Autodesk Fusion 360 part; units mm, degrees
(part 2 of 8)
  line L971 (783.8506, -24.35) -> (783.8506, -21.35)
  line L972 (783.8506, -21.35) -> (780.8506, -21.35)
  line L973 (780.8506, -21.35) -> (780.8506, -24.35)
  line L974 (780.8506, -24.35) -> (777.8506, -24.35)
  line L975 (777.8506, -24.35) -> (777.8506, -21.35)
  line L976 (777.8506, -21.35) -> (774.8506, -21.35)
  line L977 (774.8506, -21.35) -> (774.8506, -24.35)
  line L978 (774.8506, -24.35) -> (771.8506, -24.35)
  line L979 (771.8506, -24.35) -> (771.8506, -21.35)
  line L980 (771.8506, -21.35) -> (768.8506, -21.35)
  line L981 (768.8506, -21.35) -> (768.8506, -24.35)
  line L982 (768.8506, -24.35) -> (765.8506, -24.35)
  line L983 (765.8506, -24.35) -> (765.8506, -21.35)
  line L984 (765.8506, -21.35) -> (762.8506, -21.35)
  line L985 (762.8506, -21.35) -> (762.8506, -24.35)
  line L986 (762.8506, -24.35) -> (759.8506, -24.35)
  line L987 (759.8506, -24.35) -> (759.8506, -21.35)
  line L988 (759.8506, -21.35) -> (756.8506, -21.35)
  line L989 (756.8506, -21.35) -> (756.8506, -24.35)
  line L990 (756.8506, -24.35) -> (753.8506, -24.35)
  line L991 (753.8506, -24.35) -> (753.8506, -21.35)
  line L992 (753.8506, -21.35) -> (750.8506, -21.35)
  line L993 (750.8506, -21.35) -> (750.8506, -24.35)
  line L994 (750.8506, -24.35) -> (747.8506, -24.35)
  line L995 (747.8506, -24.35) -> (747.8506, -21.35)
  line L996 (747.8506, -21.35) -> (744.8506, -21.35)
  line L997 (744.8506, -21.35) -> (744.8506, -24.35)
  line L998 (744.8506, -24.35) -> (741.8506, -24.35)
  line L999 (741.8506, -24.35) -> (741.8506, -21.35)
  line L1000 (741.8506, -21.35) -> (738.8506, -21.35)
  line L1001 (738.8506, -21.35) -> (738.8506, -24.35)
  line L1002 (738.8506, -24.35) -> (735.8506, -24.35)
  line L1003 (735.8506, -24.35) -> (735.8506, -21.35)
  line L1004 (735.8506, -21.35) -> (732.8506, -21.35)
  line L1005 (732.8506, -21.35) -> (732.8506, -24.35)
  line L1006 (732.8506, -24.35) -> (729.8506, -24.35)
  line L1007 (729.8506, -24.35) -> (729.8506, -21.35)
  line L1008 (729.8506, -21.35) -> (726.8506, -21.35)
  line L1009 (726.8506, -21.35) -> (726.8506, -24.35)
  line L1010 (726.8506, -24.35) -> (723.8506, -24.35)
  line L1011 (723.8506, -24.35) -> (723.8506, -21.35)
  line L1012 (723.8506, -21.35) -> (720.8506, -21.35)
  line L1013 (720.8506, -21.35) -> (720.8506, -24.35)
  line L1014 (720.8506, -24.35) -> (717.8506, -24.35)
  line L1015 (717.8506, -24.35) -> (717.8506, -21.35)
  line L1016 (717.8506, -21.35) -> (714.8506, -21.35)
  line L1017 (714.8506, -21.35) -> (714.8506, -24.35)
  line L1018 (714.8506, -24.35) -> (711.8506, -24.35)
  line L1019 (711.8506, -24.35) -> (711.8506, -21.35)
  line L1020 (711.8506, -21.35) -> (708.8506, -21.35)
  line L1021 (708.8506, -21.35) -> (708.8506, -24.35)
  line L1022 (708.8506, -24.35) -> (705.8506, -24.35)
  line L1023 (705.8506, -24.35) -> (705.8506, -21.35)
  line L1024 (705.8506, -21.35) -> (702.8506, -21.35)
  line L1025 (702.8506, -21.35) -> (702.8506, -24.35)
  line L1026 (702.8506, -24.35) -> (699.8506, -24.35)
  line L1027 (699.8506, -24.35) -> (699.8506, -21.35)
  line L1028 (699.8506, -21.35) -> (696.8506, -21.35)
  line L1029 (696.8506, -21.35) -> (696.8506, -24.35)
  line L1030 (696.8506, -24.35) -> (693.8506, -24.35)
  line L1031 (693.8506, -24.35) -> (693.8506, -21.35)
  line L1032 (693.8506, -21.35) -> (690.8506, -21.35)
  line L1033 (690.8506, -21.35) -> (690.8506, -24.35)
  line L1034 (690.8506, -24.35) -> (687.8506, -24.35)
  line L1035 (687.8506, -24.35) -> (687.8506, -21.35)
  line L1036 (687.8506, -21.35) -> (684.8506, -21.35)
  line L1037 (684.8506, -21.35) -> (684.8506, -24.35)
  line L1038 (684.8506, -24.35) -> (681.8506, -24.35)
  line L1039 (681.8506, -24.35) -> (681.8506, -21.35)
  line L1040 (681.8506, -21.35) -> (678.8506, -21.35)
  line L1041 (678.8506, -21.35) -> (678.8506, -24.35)
  line L1042 (678.8506, -24.35) -> (675.8506, -24.35)
  line L1043 (675.8506, -24.35) -> (675.8506, -21.35)
  line L1044 (675.8506, -21.35) -> (672.8506, -21.35)
  line L1045 (672.8506, -21.35) -> (672.8506, -24.35)
  line L1046 (672.8506, -24.35) -> (669.8506, -24.35)
  line L1047 (669.8506, -24.35) -> (669.8506, -21.35)
  line L1048 (669.8506, -21.35) -> (666.8505, -21.35)
  line L1049 (666.8505, -21.35) -> (666.8505, -24.35)
  line L1050 (666.8505, -24.35) -> (663.8505, -24.35)
  line L1051 (663.8505, -24.35) -> (663.8505, -21.35)
  line L1052 (663.8505, -21.35) -> (660.8505, -21.35)
  line L1053 (660.8505, -21.35) -> (660.8505, -24.35)
  line L1054 (660.8505, -24.35) -> (657.8505, -24.35)
  line L1055 (657.8505, -24.35) -> (657.8505, -21.35)
  line L1056 (657.8505, -21.35) -> (654.8505, -21.35)
  line L1057 (654.8505, -21.35) -> (654.8505, -24.35)
  line L1058 (654.8505, -24.35) -> (651.8505, -24.35)
  line L1059 (651.8505, -24.35) -> (651.8505, -21.35)
  line L1060 (651.8505, -21.35) -> (648.8505, -21.35)
  line L1061 (648.8505, -21.35) -> (648.8505, -24.35)
  line L1062 (648.8505, -24.35) -> (645.8505, -24.35)
  line L1063 (645.8505, -24.35) -> (645.8505, -21.35)
  line L1064 (645.8505, -21.35) -> (642.1005, -21.35)
  line L1065 (642.1005, -21.35) -> (642.1005, -24.35)
  line L1066 (642.1005, -24.35) -> (641.3505, -24.35)
  line L1067 (641.3505, -24.35) -> (641.3505, -20.6)
  line L1068 (641.3505, -20.6) -> (638.3505, -20.6)
  line L1069 (638.3505, -20.6) -> (638.3505, -16.85)
  line L1070 (638.3505, -16.85) -> (641.3505, -16.85)
  line L1071 (641.3505, -16.85) -> (641.3505, -13.85)
  line L1072 (641.3505, -13.85) -> (638.3505, -13.85)
  line L1073 (638.3505, -13.85) -> (638.3505, -10.1)
  line L1074 (638.3505, -10.1) -> (641.3505, -10.1)
  line L1075 (641.3505, -10.1) -> (641.3505, -6.35)
  line L1076 (641.3505, -24.35) -> (642.1005, -24.35)
  line L1077 (642.1005, -24.35) -> (642.1005, -27.35)
  line L1078 (642.1005, -27.35) -> (645.8505, -27.35)
  line L1079 (645.8505, -27.35) -> (645.8505, -24.35)
  line L1080 (645.8505, -24.35) -> (648.8505, -24.35)
  line L1081 (648.8505, -24.35) -> (648.8505, -27.35)
  line L1082 (648.8505, -27.35) -> (651.8505, -27.35)
  line L1083 (651.8505, -27.35) -> (651.8505, -24.35)
  line L1084 (651.8505, -24.35) -> (654.8505, -24.35)
  line L1085 (654.8505, -24.35) -> (654.8505, -27.35)
  line L1086 (654.8505, -27.35) -> (657.8505, -27.35)
  line L1087 (657.8505, -27.35) -> (657.8505, -24.35)
  line L1088 (657.8505, -24.35) -> (660.8505, -24.35)
  line L1089 (660.8505, -24.35) -> (660.8505, -27.35)
  line L1090 (660.8505, -27.35) -> (663.8505, -27.35)
  line L1091 (663.8505, -27.35) -> (663.8505, -24.35)
  line L1092 (663.8505, -24.35) -> (666.8505, -24.35)
  line L1093 (666.8505, -24.35) -> (666.8505, -27.35)
  line L1094 (666.8505, -27.35) -> (669.8506, -27.35)
  line L1095 (669.8506, -27.35) -> (669.8506, -24.35)
  line L1096 (669.8506, -24.35) -> (672.8506, -24.35)
  line L1097 (672.8506, -24.35) -> (672.8506, -27.35)
  line L1098 (672.8506, -27.35) -> (675.8506, -27.35)
  line L1099 (675.8506, -27.35) -> (675.8506, -24.35)
  line L1100 (675.8506, -24.35) -> (678.8506, -24.35)
  line L1101 (678.8506, -24.35) -> (678.8506, -27.35)
  line L1102 (678.8506, -27.35) -> (681.8506, -27.35)
  line L1103 (681.8506, -27.35) -> (681.8506, -24.35)
  line L1104 (681.8506, -24.35) -> (684.8506, -24.35)
  line L1105 (684.8506, -24.35) -> (684.8506, -27.35)
  line L1106 (684.8506, -27.35) -> (687.8506, -27.35)
  line L1107 (687.8506, -27.35) -> (687.8506, -24.35)
  line L1108 (687.8506, -24.35) -> (690.8506, -24.35)
  line L1109 (690.8506, -24.35) -> (690.8506, -27.35)
  line L1110 (690.8506, -27.35) -> (693.8506, -27.35)
  line L1111 (693.8506, -27.35) -> (693.8506, -24.35)
  line L1112 (693.8506, -24.35) -> (696.8506, -24.35)
  line L1113 (696.8506, -24.35) -> (696.8506, -27.35)
  line L1114 (696.8506, -27.35) -> (699.8506, -27.35)
  line L1115 (699.8506, -27.35) -> (699.8506, -24.35)
  line L1116 (699.8506, -24.35) -> (702.8506, -24.35)
  line L1117 (702.8506, -24.35) -> (702.8506, -27.35)
  line L1118 (702.8506, -27.35) -> (705.8506, -27.35)
  line L1119 (705.8506, -27.35) -> (705.8506, -24.35)
  line L1120 (705.8506, -24.35) -> (708.8506, -24.35)
  line L1121 (708.8506, -24.35) -> (708.8506, -27.35)
  line L1122 (708.8506, -27.35) -> (711.8506, -27.35)
  line L1123 (711.8506, -27.35) -> (711.8506, -24.35)
  line L1124 (711.8506, -24.35) -> (714.8506, -24.35)
  line L1125 (714.8506, -24.35) -> (714.8506, -27.35)
  line L1126 (714.8506, -27.35) -> (717.8506, -27.35)
  line L1127 (717.8506, -27.35) -> (717.8506, -24.35)
  line L1128 (717.8506, -24.35) -> (720.8506, -24.35)
  line L1129 (720.8506, -24.35) -> (720.8506, -27.35)
  line L1130 (720.8506, -27.35) -> (723.8506, -27.35)
  line L1131 (723.8506, -27.35) -> (723.8506, -24.35)
  line L1132 (723.8506, -24.35) -> (726.8506, -24.35)
  line L1133 (726.8506, -24.35) -> (726.8506, -27.35)
  line L1134 (726.8506, -27.35) -> (729.8506, -27.35)
  line L1135 (729.8506, -27.35) -> (729.8506, -24.35)
  line L1136 (729.8506, -24.35) -> (732.8506, -24.35)
  line L1137 (732.8506, -24.35) -> (732.8506, -27.35)
  line L1138 (732.8506, -27.35) -> (735.8506, -27.35)
  line L1139 (735.8506, -27.35) -> (735.8506, -24.35)
  line L1140 (735.8506, -24.35) -> (738.8506, -24.35)
  line L1141 (738.8506, -24.35) -> (738.8506, -27.35)
  line L1142 (738.8506, -27.35) -> (741.8506, -27.35)
  line L1143 (741.8506, -27.35) -> (741.8506, -24.35)
  line L1144 (741.8506, -24.35) -> (744.8506, -24.35)
  line L1145 (744.8506, -24.35) -> (744.8506, -27.35)
  line L1146 (744.8506, -27.35) -> (747.8506, -27.35)
  line L1147 (747.8506, -27.35) -> (747.8506, -24.35)
  line L1148 (747.8506, -24.35) -> (750.8506, -24.35)
  line L1149 (750.8506, -24.35) -> (750.8506, -27.35)
  line L1150 (750.8506, -27.35) -> (753.8506, -27.35)
  line L1151 (753.8506, -27.35) -> (753.8506, -24.35)
  line L1152 (753.8506, -24.35) -> (756.8506, -24.35)
  line L1153 (756.8506, -24.35) -> (756.8506, -27.35)
  line L1154 (756.8506, -27.35) -> (759.8506, -27.35)
  line L1155 (759.8506, -27.35) -> (759.8506, -24.35)
  line L1156 (759.8506, -24.35) -> (762.8506, -24.35)
  line L1157 (762.8506, -24.35) -> (762.8506, -27.35)
  line L1158 (762.8506, -27.35) -> (765.8506, -27.35)
  line L1159 (765.8506, -27.35) -> (765.8506, -24.35)
  line L1160 (765.8506, -24.35) -> (768.8506, -24.35)
  line L1161 (768.8506, -24.35) -> (768.8506, -27.35)
  line L1162 (768.8506, -27.35) -> (771.8506, -27.35)
  line L1163 (771.8506, -27.35) -> (771.8506, -24.35)
  line L1164 (771.8506, -24.35) -> (774.8506, -24.35)
  line L1165 (774.8506, -24.35) -> (774.8506, -27.35)
  line L1166 (774.8506, -27.35) -> (777.8506, -27.35)
  line L1167 (777.8506, -27.35) -> (777.8506, -24.35)
  line L1168 (777.8506, -24.35) -> (780.8506, -24.35)
  line L1169 (780.8506, -24.35) -> (780.8506, -27.35)
  line L1170 (780.8506, -27.35) -> (783.8506, -27.35)
  line L1171 (783.8506, -27.35) -> (783.8506, -24.35)
  line L1172 (783.8506, -24.35) -> (786.8506, -24.35)
  line L1173 (786.8506, -24.35) -> (786.8506, -27.35)
  line L1174 (786.8506, -27.35) -> (790.6007, -27.35)
  line L1175 (790.6007, -27.35) -> (790.6007, -24.35)
  line L1176 (790.6007, -24.35) -> (791.3507, -24.35)
  line L1177 (791.3507, -24.35) -> (791.3507, -28.1)
  line L1178 (791.3507, -28.1) -> (794.3507, -28.1)
  line L1179 (794.3507, -28.1) -> (794.3507, -31.85)
  line L1180 (794.3507, -31.85) -> (791.3507, -31.85)
  line L1181 (791.3507, -31.85) -> (791.3507, -34.85)
  line L1182 (791.3507, -34.85) -> (794.3507, -34.85)
  line L1183 (794.3507, -34.85) -> (794.3507, -38.6)
  line L1184 (794.3507, -38.6) -> (791.3507, -38.6)
  line L1185 (791.3507, -38.6) -> (791.3507, -42.35)
  line L1186 (791.3507, -42.35) -> (790.6007, -42.35)
  line L1187 (790.6007, -42.35) -> (790.6007, -39.35)
  line L1188 (790.6007, -39.35) -> (786.8506, -39.35)
  line L1189 (786.8506, -39.35) -> (786.8506, -42.35)
  line L1190 (786.8506, -42.35) -> (783.8506, -42.35)
  line L1191 (783.8506, -42.35) -> (783.8506, -39.35)
  line L1192 (783.8506, -39.35) -> (780.8506, -39.35)
  line L1193 (780.8506, -39.35) -> (780.8506, -42.35)
  line L1194 (780.8506, -42.35) -> (777.8506, -42.35)
  line L1195 (777.8506, -42.35) -> (777.8506, -39.35)
  line L1196 (777.8506, -39.35) -> (774.8506, -39.35)
  line L1197 (774.8506, -39.35) -> (774.8506, -42.35)
  line L1198 (774.8506, -42.35) -> (771.8506, -42.35)
  line L1199 (771.8506, -42.35) -> (771.8506, -39.35)
  line L1200 (771.8506, -39.35) -> (768.8506, -39.35)
  line L1201 (768.8506, -39.35) -> (768.8506, -42.35)
  line L1202 (768.8506, -42.35) -> (765.8506, -42.35)
  line L1203 (765.8506, -42.35) -> (765.8506, -39.35)
  line L1204 (765.8506, -39.35) -> (762.8506, -39.35)
  line L1205 (762.8506, -39.35) -> (762.8506, -42.35)
  line L1206 (762.8506, -42.35) -> (759.8506, -42.35)
  line L1207 (759.8506, -42.35) -> (759.8506, -39.35)
  line L1208 (759.8506, -39.35) -> (756.8506, -39.35)
  line L1209 (756.8506, -39.35) -> (756.8506, -42.35)
  line L1210 (756.8506, -42.35) -> (753.8506, -42.35)
  line L1211 (753.8506, -42.35) -> (753.8506, -39.35)
  line L1212 (753.8506, -39.35) -> (750.8506, -39.35)
  line L1213 (750.8506, -39.35) -> (750.8506, -42.35)
  line L1214 (750.8506, -42.35) -> (747.8506, -42.35)
  line L1215 (747.8506, -42.35) -> (747.8506, -39.35)
  line L1216 (747.8506, -39.35) -> (744.8506, -39.35)
  line L1217 (744.8506, -39.35) -> (744.8506, -42.35)
  line L1218 (744.8506, -42.35) -> (741.8506, -42.35)
  line L1219 (741.8506, -42.35) -> (741.8506, -39.35)
  line L1220 (741.8506, -39.35) -> (738.8506, -39.35)
  line L1221 (738.8506, -39.35) -> (738.8506, -42.35)
  line L1222 (738.8506, -42.35) -> (735.8506, -42.35)
  line L1223 (735.8506, -42.35) -> (735.8506, -39.35)
  line L1224 (735.8506, -39.35) -> (732.8506, -39.35)
  line L1225 (732.8506, -39.35) -> (732.8506, -42.35)
  line L1226 (732.8506, -42.35) -> (729.8506, -42.35)
  line L1227 (729.8506, -42.35) -> (729.8506, -39.35)
  line L1228 (729.8506, -39.35) -> (726.8506, -39.35)
  line L1229 (726.8506, -39.35) -> (726.8506, -42.35)
  line L1230 (726.8506, -42.35) -> (723.8506, -42.35)
  line L1231 (723.8506, -42.35) -> (723.8506, -39.35)
  line L1232 (723.8506, -39.35) -> (720.8506, -39.35)
  line L1233 (720.8506, -39.35) -> (720.8506, -42.35)
  line L1234 (720.8506, -42.35) -> (717.8506, -42.35)
  line L1235 (717.8506, -42.35) -> (717.8506, -39.35)
  line L1236 (717.8506, -39.35) -> (714.8506, -39.35)
  line L1237 (714.8506, -39.35) -> (714.8506, -42.35)
  line L1238 (714.8506, -42.35) -> (711.8506, -42.35)
  line L1239 (711.8506, -42.35) -> (711.8506, -39.35)
  line L1240 (711.8506, -39.35) -> (708.8506, -39.35)
  line L1241 (708.8506, -39.35) -> (708.8506, -42.35)
  line L1242 (708.8506, -42.35) -> (705.8506, -42.35)
  line L1243 (705.8506, -42.35) -> (705.8506, -39.35)
  line L1244 (705.8506, -39.35) -> (702.8506, -39.35)
  line L1245 (702.8506, -39.35) -> (702.8506, -42.35)
  line L1246 (702.8506, -42.35) -> (699.8506, -42.35)
  line L1247 (699.8506, -42.35) -> (699.8506, -39.35)
  line L1248 (699.8506, -39.35) -> (696.8506, -39.35)
  line L1249 (696.8506, -39.35) -> (696.8506, -42.35)
  line L1250 (696.8506, -42.35) -> (693.8506, -42.35)
  line L1251 (693.8506, -42.35) -> (693.8506, -39.35)
  line L1252 (693.8506, -39.35) -> (690.8506, -39.35)
  line L1253 (690.8506, -39.35) -> (690.8506, -42.35)
  line L1254 (690.8506, -42.35) -> (687.8506, -42.35)
  line L1255 (687.8506, -42.35) -> (687.8506, -39.35)
  line L1256 (687.8506, -39.35) -> (684.8506, -39.35)
  line L1257 (684.8506, -39.35) -> (684.8506, -42.35)
  line L1258 (684.8506, -42.35) -> (681.8506, -42.35)
  line L1259 (681.8506, -42.35) -> (681.8506, -39.35)
  line L1260 (681.8506, -39.35) -> (678.8506, -39.35)
  line L1261 (678.8506, -39.35) -> (678.8506, -42.35)
  line L1262 (678.8506, -42.35) -> (675.8506, -42.35)
  line L1263 (675.8506, -42.35) -> (675.8506, -39.35)
  line L1264 (675.8506, -39.35) -> (672.8506, -39.35)
  line L1265 (672.8506, -39.35) -> (672.8506, -42.35)
  line L1266 (672.8506, -42.35) -> (669.8506, -42.35)
  line L1267 (669.8506, -42.35) -> (669.8506, -39.35)
  line L1268 (669.8506, -39.35) -> (666.8505, -39.35)
  line L1269 (666.8505, -39.35) -> (666.8505, -42.35)
  line L1270 (666.8505, -42.35) -> (663.8505, -42.35)
  line L1271 (663.8505, -42.35) -> (663.8505, -39.35)
  line L1272 (663.8505, -39.35) -> (660.8505, -39.35)
  line L1273 (660.8505, -39.35) -> (660.8505, -42.35)
  line L1274 (660.8505, -42.35) -> (657.8505, -42.35)
  line L1275 (657.8505, -42.35) -> (657.8505, -39.35)
  line L1276 (657.8505, -39.35) -> (654.8505, -39.35)
  line L1277 (654.8505, -39.35) -> (654.8505, -42.35)
  line L1278 (654.8505, -42.35) -> (651.8505, -42.35)
  line L1279 (651.8505, -42.35) -> (651.8505, -39.35)
  line L1280 (651.8505, -39.35) -> (648.8505, -39.35)
  line L1281 (648.8505, -39.35) -> (648.8505, -42.35)
  line L1282 (648.8505, -42.35) -> (645.8505, -42.35)
  line L1283 (645.8505, -42.35) -> (645.8505, -39.35)
  line L1284 (645.8505, -39.35) -> (642.1005, -39.35)
  line L1285 (642.1005, -39.35) -> (642.1005, -42.35)
  line L1286 (642.1005, -42.35) -> (641.3505, -42.35)
  line L1287 (641.3505, -42.35) -> (641.3505, -38.6)
  line L1288 (641.3505, -38.6) -> (638.3505, -38.6)
  line L1289 (638.3505, -38.6) -> (638.3505, -34.85)
  line L1290 (638.3505, -34.85) -> (641.3505, -34.85)
  line L1291 (641.3505, -34.85) -> (641.3505, -31.85)
  line L1292 (641.3505, -31.85) -> (638.3505, -31.85)
  line L1293 (638.3505, -31.85) -> (638.3505, -28.1)
  line L1294 (638.3505, -28.1) -> (641.3505, -28.1)
  line L1295 (641.3505, -28.1) -> (641.3505, -24.35)
  line L1296 (9.35, -27.35) -> (11.1, -27.35)
  line L1297 (11.1, -27.35) -> (11.1, -24.35)
  line L1298 (11.1, -24.35) -> (15.85, -24.35)
  line L1299 (15.85, -24.35) -> (15.85, -27.35)
  line L1300 (15.85, -27.35) -> (18.85, -27.35)
  line L1301 (18.85, -27.35) -> (18.85, -24.35)
  line L1302 (18.85, -24.35) -> (21.85, -24.35)
  line L1303 (21.85, -24.35) -> (21.85, -27.35)
  line L1304 (21.85, -27.35) -> (24.85, -27.35)
  line L1305 (24.85, -27.35) -> (24.85, -24.35)
  line L1306 (24.85, -24.35) -> (27.85, -24.35)
  line L1307 (27.85, -24.35) -> (27.85, -27.35)
  line L1308 (27.85, -27.35) -> (30.85, -27.35)
  line L1309 (30.85, -27.35) -> (30.85, -24.35)
  line L1310 (30.85, -24.35) -> (33.85, -24.35)
  line L1311 (33.85, -24.35) -> (33.85, -27.35)
  line L1312 (33.85, -27.35) -> (36.85, -27.35)
  line L1313 (36.85, -27.35) -> (36.85, -24.35)
  line L1314 (36.85, -24.35) -> (39.85, -24.35)
  line L1315 (39.85, -24.35) -> (39.85, -27.35)
  line L1316 (39.85, -27.35) -> (42.85, -27.35)
  line L1317 (42.85, -27.35) -> (42.85, -24.35)
  line L1318 (42.85, -24.35) -> (45.85, -24.35)
  line L1319 (45.85, -24.35) -> (45.85, -27.35)
  line L1320 (45.85, -27.35) -> (48.85, -27.35)
  line L1321 (48.85, -27.35) -> (48.85, -24.35)
  line L1322 (48.85, -24.35) -> (51.85, -24.35)
  line L1323 (51.85, -24.35) -> (51.85, -27.35)
  line L1324 (51.85, -27.35) -> (54.85, -27.35)
  line L1325 (54.85, -27.35) -> (54.85, -24.35)
  line L1326 (54.85, -24.35) -> (57.85, -24.35)
  line L1327 (57.85, -24.35) -> (57.85, -27.35)
  line L1328 (57.85, -27.35) -> (60.8501, -27.35)
  line L1329 (60.8501, -27.35) -> (60.8501, -24.35)
  line L1330 (60.8501, -24.35) -> (63.8501, -24.35)
  line L1331 (63.8501, -24.35) -> (63.8501, -27.35)
  line L1332 (63.8501, -27.35) -> (66.8501, -27.35)
  line L1333 (66.8501, -27.35) -> (66.8501, -24.35)
  line L1334 (66.8501, -24.35) -> (69.8501, -24.35)
  line L1335 (69.8501, -24.35) -> (69.8501, -27.35)
  line L1336 (69.8501, -27.35) -> (72.8501, -27.35)
  line L1337 (72.8501, -27.35) -> (72.8501, -24.35)
  line L1338 (72.8501, -24.35) -> (75.8501, -24.35)
  line L1339 (75.8501, -24.35) -> (75.8501, -27.35)
  line L1340 (75.8501, -27.35) -> (78.8501, -27.35)
  line L1341 (78.8501, -27.35) -> (78.8501, -24.35)
  line L1342 (78.8501, -24.35) -> (81.8501, -24.35)
  line L1343 (81.8501, -24.35) -> (81.8501, -27.35)
  line L1344 (81.8501, -27.35) -> (84.8501, -27.35)
  line L1345 (84.8501, -27.35) -> (84.8501, -24.35)
  line L1346 (84.8501, -24.35) -> (87.8501, -24.35)
  line L1347 (87.8501, -24.35) -> (87.8501, -27.35)
  line L1348 (87.8501, -27.35) -> (90.8501, -27.35)
  line L1349 (90.8501, -27.35) -> (90.8501, -24.35)
  line L1350 (90.8501, -24.35) -> (93.8501, -24.35)
  line L1351 (93.8501, -24.35) -> (93.8501, -27.35)
  line L1352 (93.8501, -27.35) -> (96.8501, -27.35)
  line L1353 (96.8501, -27.35) -> (96.8501, -24.35)
  line L1354 (96.8501, -24.35) -> (99.8501, -24.35)
  line L1355 (99.8501, -24.35) -> (99.8501, -27.35)
  line L1356 (99.8501, -27.35) -> (102.8501, -27.35)
  line L1357 (102.8501, -27.35) -> (102.8501, -24.35)
  line L1358 (102.8501, -24.35) -> (105.8501, -24.35)
  line L1359 (105.8501, -24.35) -> (105.8501, -27.35)
  line L1360 (105.8501, -27.35) -> (108.8501, -27.35)
  line L1361 (108.8501, -27.35) -> (108.8501, -24.35)
  line L1362 (108.8501, -24.35) -> (111.8501, -24.35)
  line L1363 (111.8501, -24.35) -> (111.8501, -27.35)
  line L1364 (111.8501, -27.35) -> (114.8501, -27.35)
  line L1365 (114.8501, -27.35) -> (114.8501, -24.35)
  line L1366 (114.8501, -24.35) -> (117.8501, -24.35)
  line L1367 (117.8501, -24.35) -> (117.8501, -27.35)
  line L1368 (117.8501, -27.35) -> (120.8501, -27.35)
  line L1369 (120.8501, -27.35) -> (120.8501, -24.35)
  line L1370 (120.8501, -24.35) -> (123.8501, -24.35)
  line L1371 (123.8501, -24.35) -> (123.8501, -27.35)
  line L1372 (123.8501, -27.35) -> (126.8501, -27.35)
  line L1373 (126.8501, -27.35) -> (126.8501, -24.35)
  line L1374 (126.8501, -24.35) -> (129.8501, -24.35)
  line L1375 (129.8501, -24.35) -> (129.8501, -27.35)
  line L1376 (129.8501, -27.35) -> (132.8501, -27.35)
  line L1377 (132.8501, -27.35) -> (132.8501, -24.35)
  line L1378 (132.8501, -24.35) -> (135.8501, -24.35)
  line L1379 (135.8501, -24.35) -> (135.8501, -27.35)
  line L1380 (135.8501, -27.35) -> (138.8501, -27.35)
  line L1381 (138.8501, -27.35) -> (138.8501, -24.35)
  line L1382 (138.8501, -24.35) -> (141.8501, -24.35)
  line L1383 (141.8501, -24.35) -> (141.8501, -27.35)
  line L1384 (141.8501, -27.35) -> (144.8501, -27.35)
  line L1385 (144.8501, -27.35) -> (144.8501, -24.35)
  line L1386 (144.8501, -24.35) -> (147.8501, -24.35)
  line L1387 (147.8501, -24.35) -> (147.8501, -27.35)
  line L1388 (147.8501, -27.35) -> (150.8501, -27.35)
  line L1389 (150.8501, -27.35) -> (150.8501, -24.35)
  line L1390 (150.8501, -24.35) -> (153.8501, -24.35)
  line L1391 (153.8501, -24.35) -> (153.8501, -27.35)
  line L1392 (153.8501, -27.35) -> (156.8501, -27.35)
  line L1393 (156.8501, -27.35) -> (156.8501, -24.35)
  line L1394 (156.8501, -24.35) -> (159.8501, -24.35)
  line L1395 (159.8501, -24.35) -> (159.8501, -27.35)
  line L1396 (159.8501, -27.35) -> (162.8501, -27.35)
  line L1397 (162.8501, -27.35) -> (162.8501, -24.35)
  line L1398 (162.8501, -24.35) -> (165.8501, -24.35)
  line L1399 (165.8501, -24.35) -> (165.8501, -27.35)
  line L1400 (165.8501, -27.35) -> (168.8501, -27.35)
  line L1401 (168.8501, -27.35) -> (168.8501, -24.35)
  line L1402 (168.8501, -24.35) -> (171.8501, -24.35)
  line L1403 (171.8501, -24.35) -> (171.8501, -27.35)
  line L1404 (171.8501, -27.35) -> (174.8501, -27.35)
  line L1405 (174.8501, -27.35) -> (174.8501, -24.35)
  line L1406 (174.8501, -24.35) -> (177.8501, -24.35)
  line L1407 (177.8501, -24.35) -> (177.8501, -27.35)
  line L1408 (177.8501, -27.35) -> (180.8501, -27.35)
  line L1409 (180.8501, -27.35) -> (180.8501, -24.35)
  line L1410 (180.8501, -24.35) -> (183.8502, -24.35)
  line L1411 (183.8502, -24.35) -> (183.8502, -27.35)
  line L1412 (183.8502, -27.35) -> (186.8502, -27.35)
  line L1413 (186.8502, -27.35) -> (186.8502, -24.35)
  line L1414 (186.8502, -24.35) -> (189.8502, -24.35)
  line L1415 (189.8502, -24.35) -> (189.8502, -27.35)
  line L1416 (189.8502, -27.35) -> (192.8502, -27.35)
  line L1417 (192.8502, -27.35) -> (192.8502, -24.35)
  line L1418 (192.8502, -24.35) -> (195.8502, -24.35)
  line L1419 (195.8502, -24.35) -> (195.8502, -27.35)
  line L1420 (195.8502, -27.35) -> (198.8502, -27.35)
  line L1421 (198.8502, -27.35) -> (198.8502, -24.35)
  line L1422 (198.8502, -24.35) -> (201.8502, -24.35)
  line L1423 (201.8502, -24.35) -> (201.8502, -27.35)
  line L1424 (201.8502, -27.35) -> (204.8502, -27.35)
  line L1425 (204.8502, -27.35) -> (204.8502, -24.35)
  line L1426 (204.8502, -24.35) -> (207.8502, -24.35)
  line L1427 (207.8502, -24.35) -> (207.8502, -27.35)
  line L1428 (207.8502, -27.35) -> (210.8502, -27.35)
  line L1429 (210.8502, -27.35) -> (210.8502, -24.35)
  line L1430 (210.8502, -24.35) -> (213.8502, -24.35)
  line L1431 (213.8502, -24.35) -> (213.8502, -27.35)
  line L1432 (213.8502, -27.35) -> (216.8502, -27.35)
  line L1433 (216.8502, -27.35) -> (216.8502, -24.35)
  line L1434 (216.8502, -24.35) -> (219.8502, -24.35)
  line L1435 (219.8502, -24.35) -> (219.8502, -27.35)
  line L1436 (219.8502, -27.35) -> (222.8502, -27.35)
  line L1437 (222.8502, -27.35) -> (222.8502, -24.35)
  line L1438 (222.8502, -24.35) -> (225.8502, -24.35)
  line L1439 (225.8502, -24.35) -> (225.8502, -27.35)
  line L1440 (225.8502, -27.35) -> (228.8502, -27.35)
  line L1441 (228.8502, -27.35) -> (228.8502, -24.35)
  line L1442 (228.8502, -24.35) -> (231.8502, -24.35)
  line L1443 (231.8502, -24.35) -> (231.8502, -27.35)
  line L1444 (231.8502, -27.35) -> (234.8502, -27.35)
  line L1445 (234.8502, -27.35) -> (234.8502, -24.35)
  line L1446 (234.8502, -24.35) -> (237.8502, -24.35)
  line L1447 (237.8502, -24.35) -> (237.8502, -27.35)
  line L1448 (237.8502, -27.35) -> (240.8502, -27.35)
  line L1449 (240.8502, -27.35) -> (240.8502, -24.35)
  line L1450 (240.8502, -24.35) -> (243.8502, -24.35)
  line L1451 (243.8502, -24.35) -> (243.8502, -27.35)
  line L1452 (243.8502, -27.35) -> (246.8502, -27.35)
  line L1453 (246.8502, -27.35) -> (246.8502, -24.35)
  line L1454 (246.8502, -24.35) -> (249.8502, -24.35)
  line L1455 (249.8502, -24.35) -> (249.8502, -27.35)
  line L1456 (249.8502, -27.35) -> (252.8502, -27.35)
  line L1457 (252.8502, -27.35) -> (252.8502, -24.35)
  line L1458 (252.8502, -24.35) -> (255.8502, -24.35)
  line L1459 (255.8502, -24.35) -> (255.8502, -27.35)
  line L1460 (255.8502, -27.35) -> (258.8502, -27.35)
  line L1461 (258.8502, -27.35) -> (258.8502, -24.35)
  line L1462 (258.8502, -24.35) -> (261.8502, -24.35)
  line L1463 (261.8502, -24.35) -> (261.8502, -27.35)
  line L1464 (261.8502, -27.35) -> (264.8502, -27.35)
  line L1465 (264.8502, -27.35) -> (264.8502, -24.35)
  line L1466 (264.8502, -24.35) -> (267.8502, -24.35)
  line L1467 (267.8502, -24.35) -> (267.8502, -27.35)
  line L1468 (267.8502, -27.35) -> (270.8502, -27.35)
  line L1469 (270.8502, -27.35) -> (270.8502, -24.35)
  line L1470 (270.8502, -24.35) -> (273.8502, -24.35)
  line L1471 (273.8502, -24.35) -> (273.8502, -27.35)
  line L1472 (273.8502, -27.35) -> (276.8502, -27.35)
  line L1473 (276.8502, -27.35) -> (276.8502, -24.35)
  line L1474 (276.8502, -24.35) -> (279.8502, -24.35)
  line L1475 (279.8502, -24.35) -> (279.8502, -27.35)
  line L1476 (279.8502, -27.35) -> (282.8502, -27.35)
  line L1477 (282.8502, -27.35) -> (282.8502, -24.35)
  line L1478 (282.8502, -24.35) -> (285.8502, -24.35)
  line L1479 (285.8502, -24.35) -> (285.8502, -27.35)
  line L1480 (285.8502, -27.35) -> (288.8502, -27.35)
  line L1481 (288.8502, -27.35) -> (288.8502, -24.35)
  line L1482 (288.8502, -24.35) -> (291.8502, -24.35)
  line L1483 (291.8502, -24.35) -> (291.8502, -27.35)
  line L1484 (291.8502, -27.35) -> (294.8502, -27.35)
  line L1485 (294.8502, -27.35) -> (294.8502, -24.35)
  line L1486 (294.8502, -24.35) -> (297.8502, -24.35)
  line L1487 (297.8502, -24.35) -> (297.8502, -27.35)
  line L1488 (297.8502, -27.35) -> (300.8502, -27.35)
  line L1489 (300.8502, -27.35) -> (300.8502, -24.35)
  line L1490 (300.8502, -24.35) -> (303.8502, -24.35)
  line L1491 (303.8502, -24.35) -> (303.8502, -27.35)
  line L1492 (303.8502, -27.35) -> (306.8503, -27.35)
  line L1493 (306.8503, -27.35) -> (306.8503, -24.35)
  line L1494 (306.8503, -24.35) -> (309.8503, -24.35)
  line L1495 (309.8503, -24.35) -> (309.8503, -27.35)
  line L1496 (309.8503, -27.35) -> (312.8503, -27.35)
  line L1497 (312.8503, -27.35) -> (312.8503, -24.35)
  line L1498 (312.8503, -24.35) -> (317.6003, -24.35)
  line L1499 (317.6003, -24.35) -> (317.6003, -27.35)
  line L1500 (317.6003, -27.35) -> (319.3503, -27.35)
  line L1501 (319.3503, -27.35) -> (319.3503, -28.1)
  line L1502 (319.3503, -28.1) -> (322.3503, -28.1)
  line L1503 (322.3503, -28.1) -> (322.3503, -31.85)
  line L1504 (322.3503, -31.85) -> (319.3503, -31.85)
  line L1505 (319.3503, -31.85) -> (319.3503, -34.85)
  line L1506 (319.3503, -34.85) -> (322.3503, -34.85)
  line L1507 (322.3503, -34.85) -> (322.3503, -37.85)
  line L1508 (322.3503, -37.85) -> (319.3503, -37.85)
  line L1509 (319.3503, -37.85) -> (319.3503, -40.85)
  line L1510 (319.3503, -40.85) -> (322.3503, -40.85)
  line L1511 (322.3503, -40.85) -> (322.3503, -43.85)
  line L1512 (322.3503, -43.85) -> (319.3503, -43.85)
  line L1513 (319.3503, -43.85) -> (319.3503, -46.85)
  line L1514 (319.3503, -46.85) -> (322.3503, -46.85)
  line L1515 (322.3503, -46.85) -> (322.3503, -49.85)
  line L1516 (322.3503, -49.85) -> (319.3503, -49.85)
  line L1517 (319.3503, -49.85) -> (319.3503, -52.85)
  line L1518 (319.3503, -52.85) -> (322.3503, -52.85)
  line L1519 (322.3503, -52.85) -> (322.3503, -55.85)
  line L1520 (322.3503, -55.85) -> (319.3503, -55.85)
  line L1521 (319.3503, -55.85) -> (319.3503, -58.85)
  line L1522 (319.3503, -58.85) -> (322.3503, -58.85)
  line L1523 (322.3503, -58.85) -> (322.3503, -61.8501)
  line L1524 (322.3503, -61.8501) -> (319.3503, -61.8501)
  line L1525 (319.3503, -61.8501) -> (319.3503, -64.8501)
  line L1526 (319.3503, -64.8501) -> (322.3503, -64.8501)
  line L1527 (322.3503, -64.8501) -> (322.3503, -67.8501)
  line L1528 (322.3503, -67.8501) -> (319.3503, -67.8501)
  line L1529 (319.3503, -67.8501) -> (319.3503, -70.8501)
  line L1530 (319.3503, -70.8501) -> (322.3503, -70.8501)
  line L1531 (322.3503, -70.8501) -> (322.3503, -73.8501)
  line L1532 (322.3503, -73.8501) -> (319.3503, -73.8501)
  line L1533 (319.3503, -73.8501) -> (319.3503, -76.8501)
  line L1534 (319.3503, -76.8501) -> (322.3503, -76.8501)
  line L1535 (322.3503, -76.8501) -> (322.3503, -79.8501)
  line L1536 (322.3503, -79.8501) -> (319.3503, -79.8501)
  line L1537 (319.3503, -79.8501) -> (319.3503, -82.8501)
  line L1538 (319.3503, -82.8501) -> (322.3503, -82.8501)
  line L1539 (322.3503, -82.8501) -> (322.3503, -85.8501)
  line L1540 (322.3503, -85.8501) -> (319.3503, -85.8501)
  line L1541 (319.3503, -85.8501) -> (319.3503, -88.8501)
  line L1542 (319.3503, -88.8501) -> (322.3503, -88.8501)
  line L1543 (322.3503, -88.8501) -> (322.3503, -91.8501)
  line L1544 (322.3503, -91.8501) -> (319.3503, -91.8501)
  line L1545 (319.3503, -91.8501) -> (319.3503, -94.8501)
  line L1546 (319.3503, -94.8501) -> (322.3503, -94.8501)
  line L1547 (322.3503, -94.8501) -> (322.3503, -97.8501)
  line L1548 (322.3503, -97.8501) -> (319.3503, -97.8501)
  line L1549 (319.3503, -97.8501) -> (319.3503, -100.8501)
  line L1550 (319.3503, -100.8501) -> (322.3503, -100.8501)
  line L1551 (322.3503, -100.8501) -> (322.3503, -103.8501)
  line L1552 (322.3503, -103.8501) -> (319.3503, -103.8501)
  line L1553 (319.3503, -103.8501) -> (319.3503, -106.8501)
  line L1554 (319.3503, -106.8501) -> (322.3503, -106.8501)
  line L1555 (322.3503, -106.8501) -> (322.3503, -109.8501)
  line L1556 (322.3503, -109.8501) -> (319.3503, -109.8501)
  line L1557 (319.3503, -109.8501) -> (319.3503, -112.8501)
  line L1558 (319.3503, -112.8501) -> (322.3503, -112.8501)
  line L1559 (322.3503, -112.8501) -> (322.3503, -115.8501)
  line L1560 (322.3503, -115.8501) -> (319.3503, -115.8501)
  line L1561 (319.3503, -115.8501) -> (319.3503, -118.8501)
  line L1562 (319.3503, -118.8501) -> (322.3503, -118.8501)
  line L1563 (322.3503, -118.8501) -> (322.3503, -121.8501)
  line L1564 (322.3503, -121.8501) -> (319.3503, -121.8501)
  line L1565 (319.3503, -121.8501) -> (319.3503, -124.8501)
  line L1566 (319.3503, -124.8501) -> (322.3503, -124.8501)
  line L1567 (322.3503, -124.8501) -> (322.3503, -127.8501)
  line L1568 (322.3503, -127.8501) -> (319.3503, -127.8501)
  line L1569 (319.3503, -127.8501) -> (319.3503, -130.8501)
  line L1570 (319.3503, -130.8501) -> (322.3503, -130.8501)
  line L1571 (322.3503, -130.8501) -> (322.3503, -133.8501)
  line L1572 (322.3503, -133.8501) -> (319.3503, -133.8501)
  line L1573 (319.3503, -133.8501) -> (319.3503, -136.8501)
  line L1574 (319.3503, -136.8501) -> (322.3503, -136.8501)
  line L1575 (322.3503, -136.8501) -> (322.3503, -139.8501)
  line L1576 (322.3503, -139.8501) -> (319.3503, -139.8501)
  line L1577 (319.3503, -139.8501) -> (319.3503, -142.8501)
  line L1578 (319.3503, -142.8501) -> (322.3503, -142.8501)
  line L1579 (322.3503, -142.8501) -> (322.3503, -145.8501)
  line L1580 (322.3503, -145.8501) -> (319.3503, -145.8501)
  line L1581 (319.3503, -145.8501) -> (319.3503, -148.8501)
  line L1582 (319.3503, -148.8501) -> (322.3503, -148.8501)
  line L1583 (322.3503, -148.8501) -> (322.3503, -151.8501)
  line L1584 (322.3503, -151.8501) -> (319.3503, -151.8501)
  line L1585 (319.3503, -151.8501) -> (319.3503, -154.8501)
  line L1586 (319.3503, -154.8501) -> (322.3503, -154.8501)
  line L1587 (322.3503, -154.8501) -> (322.3503, -157.8501)
  line L1588 (322.3503, -157.8501) -> (319.3503, -157.8501)
  line L1589 (319.3503, -157.8501) -> (319.3503, -160.8501)
  line L1590 (319.3503, -160.8501) -> (322.3503, -160.8501)
  line L1591 (322.3503, -160.8501) -> (322.3503, -163.8501)
  line L1592 (322.3503, -163.8501) -> (319.3503, -163.8501)
  line L1593 (319.3503, -163.8501) -> (319.3503, -166.8501)
  line L1594 (319.3503, -166.8501) -> (322.3503, -166.8501)
  line L1595 (322.3503, -166.8501) -> (322.3503, -169.8501)
  line L1596 (322.3503, -169.8501) -> (319.3503, -169.8501)
  line L1597 (319.3503, -169.8501) -> (319.3503, -172.8501)
  line L1598 (319.3503, -172.8501) -> (322.3503, -172.8501)
  line L1599 (322.3503, -172.8501) -> (322.3503, -176.6001)
  line L1600 (322.3503, -176.6001) -> (319.3503, -176.6001)
  line L1601 (319.3503, -176.6001) -> (319.3503, -177.3501)
  line L1602 (319.3503, -177.3501) -> (317.6003, -177.3501)
  line L1603 (317.6003, -177.3501) -> (317.6003, -180.3501)
  line L1604 (317.6003, -180.3501) -> (312.8503, -180.3501)
  line L1605 (312.8503, -180.3501) -> (312.8503, -177.3501)
  line L1606 (312.8503, -177.3501) -> (309.8503, -177.3501)
  line L1607 (309.8503, -177.3501) -> (309.8503, -180.3501)
  line L1608 (309.8503, -180.3501) -> (306.8503, -180.3501)
  line L1609 (306.8503, -180.3501) -> (306.8503, -177.3501)
  line L1610 (306.8503, -177.3501) -> (303.8502, -177.3501)
  line L1611 (303.8502, -177.3501) -> (303.8502, -180.3501)
  line L1612 (303.8502, -180.3501) -> (300.8502, -180.3501)
  line L1613 (300.8502, -180.3501) -> (300.8502, -177.3501)
  line L1614 (300.8502, -177.3501) -> (297.8502, -177.3501)
  line L1615 (297.8502, -177.3501) -> (297.8502, -180.3501)
  line L1616 (297.8502, -180.3501) -> (294.8502, -180.3501)
  line L1617 (294.8502, -180.3501) -> (294.8502, -177.3501)
  line L1618 (294.8502, -177.3501) -> (291.8502, -177.3501)
  line L1619 (291.8502, -177.3501) -> (291.8502, -180.3501)
  line L1620 (291.8502, -180.3501) -> (288.8502, -180.3501)
  line L1621 (288.8502, -180.3501) -> (288.8502, -177.3501)
  line L1622 (288.8502, -177.3501) -> (285.8502, -177.3501)
  line L1623 (285.8502, -177.3501) -> (285.8502, -180.3501)
  line L1624 (285.8502, -180.3501) -> (282.8502, -180.3501)
  line L1625 (282.8502, -180.3501) -> (282.8502, -177.3501)
  line L1626 (282.8502, -177.3501) -> (279.8502, -177.3501)
  line L1627 (279.8502, -177.3501) -> (279.8502, -180.3501)
  line L1628 (279.8502, -180.3501) -> (276.8502, -180.3501)
  line L1629 (276.8502, -180.3501) -> (276.8502, -177.3501)
  line L1630 (276.8502, -177.3501) -> (273.8502, -177.3501)
  line L1631 (273.8502, -177.3501) -> (273.8502, -180.3501)
  line L1632 (273.8502, -180.3501) -> (270.8502, -180.3501)
  line L1633 (270.8502, -180.3501) -> (270.8502, -177.3501)
  line L1634 (270.8502, -177.3501) -> (267.8502, -177.3501)
  line L1635 (267.8502, -177.3501) -> (267.8502, -180.3501)
  line L1636 (267.8502, -180.3501) -> (264.8502, -180.3501)
  line L1637 (264.8502, -180.3501) -> (264.8502, -177.3501)
  line L1638 (264.8502, -177.3501) -> (261.8502, -177.3501)
  line L1639 (261.8502, -177.3501) -> (261.8502, -180.3501)
  line L1640 (261.8502, -180.3501) -> (258.8502, -180.3501)
  line L1641 (258.8502, -180.3501) -> (258.8502, -177.3501)
  line L1642 (258.8502, -177.3501) -> (255.8502, -177.3501)
  line L1643 (255.8502, -177.3501) -> (255.8502, -180.3501)
  line L1644 (255.8502, -180.3501) -> (252.8502, -180.3501)
  line L1645 (252.8502, -180.3501) -> (252.8502, -177.3501)
  line L1646 (252.8502, -177.3501) -> (249.8502, -177.3501)
  line L1647 (249.8502, -177.3501) -> (249.8502, -180.3501)
  line L1648 (249.8502, -180.3501) -> (246.8502, -180.3501)
  line L1649 (246.8502, -180.3501) -> (246.8502, -177.3501)
  line L1650 (246.8502, -177.3501) -> (243.8502, -177.3501)
  line L1651 (243.8502, -177.3501) -> (243.8502, -180.3501)
  line L1652 (243.8502, -180.3501) -> (240.8502, -180.3501)
  line L1653 (240.8502, -180.3501) -> (240.8502, -177.3501)
  line L1654 (240.8502, -177.3501) -> (237.8502, -177.3501)
  line L1655 (237.8502, -177.3501) -> (237.8502, -180.3501)
  line L1656 (237.8502, -180.3501) -> (234.8502, -180.3501)
  line L1657 (234.8502, -180.3501) -> (234.8502, -177.3501)
  line L1658 (234.8502, -177.3501) -> (231.8502, -177.3501)
  line L1659 (231.8502, -177.3501) -> (231.8502, -180.3501)
  line L1660 (231.8502, -180.3501) -> (228.8502, -180.3501)
  line L1661 (228.8502, -180.3501) -> (228.8502, -177.3501)
  line L1662 (228.8502, -177.3501) -> (225.8502, -177.3501)
  line L1663 (225.8502, -177.3501) -> (225.8502, -180.3501)
  line L1664 (225.8502, -180.3501) -> (222.8502, -180.3501)
  line L1665 (222.8502, -180.3501) -> (222.8502, -177.3501)
  line L1666 (222.8502, -177.3501) -> (219.8502, -177.3501)
  line L1667 (219.8502, -177.3501) -> (219.8502, -180.3501)
  line L1668 (219.8502, -180.3501) -> (216.8502, -180.3501)
  line L1669 (216.8502, -180.3501) -> (216.8502, -177.3501)
  line L1670 (216.8502, -177.3501) -> (213.8502, -177.3501)
  line L1671 (213.8502, -177.3501) -> (213.8502, -180.3501)
  line L1672 (213.8502, -180.3501) -> (210.8502, -180.3501)
  line L1673 (210.8502, -180.3501) -> (210.8502, -177.3501)
  line L1674 (210.8502, -177.3501) -> (207.8502, -177.3501)
  line L1675 (207.8502, -177.3501) -> (207.8502, -180.3501)
  line L1676 (207.8502, -180.3501) -> (204.8502, -180.3501)
  line L1677 (204.8502, -180.3501) -> (204.8502, -177.3501)
  line L1678 (204.8502, -177.3501) -> (201.8502, -177.3501)
  line L1679 (201.8502, -177.3501) -> (201.8502, -180.3501)
  line L1680 (201.8502, -180.3501) -> (198.8502, -180.3501)
  line L1681 (198.8502, -180.3501) -> (198.8502, -177.3501)
  line L1682 (198.8502, -177.3501) -> (195.8502, -177.3501)
  line L1683 (195.8502, -177.3501) -> (195.8502, -180.3501)
  line L1684 (195.8502, -180.3501) -> (192.8502, -180.3501)
  line L1685 (192.8502, -180.3501) -> (192.8502, -177.3501)
  line L1686 (192.8502, -177.3501) -> (189.8502, -177.3501)
  line L1687 (189.8502, -177.3501) -> (189.8502, -180.3501)
  line L1688 (189.8502, -180.3501) -> (186.8502, -180.3501)
  line L1689 (186.8502, -180.3501) -> (186.8502, -177.3501)
  line L1690 (186.8502, -177.3501) -> (183.8502, -177.3501)
  line L1691 (183.8502, -177.3501) -> (183.8502, -180.3501)
  line L1692 (183.8502, -180.3501) -> (180.8501, -180.3501)
  line L1693 (180.8501, -180.3501) -> (180.8501, -177.3501)
  line L1694 (180.8501, -177.3501) -> (177.8501, -177.3501)
  line L1695 (177.8501, -177.3501) -> (177.8501, -180.3501)
  line L1696 (177.8501, -180.3501) -> (174.8501, -180.3501)
  line L1697 (174.8501, -180.3501) -> (174.8501, -177.3501)
  line L1698 (174.8501, -177.3501) -> (171.8501, -177.3501)
  line L1699 (171.8501, -177.3501) -> (171.8501, -180.3501)
  line L1700 (171.8501, -180.3501) -> (168.8501, -180.3501)
  line L1701 (168.8501, -180.3501) -> (168.8501, -177.3501)
  line L1702 (168.8501, -177.3501) -> (165.8501, -177.3501)
  line L1703 (165.8501, -177.3501) -> (165.8501, -180.3501)
  line L1704 (165.8501, -180.3501) -> (162.8501, -180.3501)
  line L1705 (162.8501, -180.3501) -> (162.8501, -177.3501)
  line L1706 (162.8501, -177.3501) -> (159.8501, -177.3501)
  line L1707 (159.8501, -177.3501) -> (159.8501, -180.3501)
  line L1708 (159.8501, -180.3501) -> (156.8501, -180.3501)
  line L1709 (156.8501, -180.3501) -> (156.8501, -177.3501)
  line L1710 (156.8501, -177.3501) -> (153.8501, -177.3501)
  line L1711 (153.8501, -177.3501) -> (153.8501, -180.3501)
  line L1712 (153.8501, -180.3501) -> (150.8501, -180.3501)
  line L1713 (150.8501, -180.3501) -> (150.8501, -177.3501)
  line L1714 (150.8501, -177.3501) -> (147.8501, -177.3501)
  line L1715 (147.8501, -177.3501) -> (147.8501, -180.3501)
  line L1716 (147.8501, -180.3501) -> (144.8501, -180.3501)
  line L1717 (144.8501, -180.3501) -> (144.8501, -177.3501)
  line L1718 (144.8501, -177.3501) -> (141.8501, -177.3501)
  line L1719 (141.8501, -177.3501) -> (141.8501, -180.3501)
  line L1720 (141.8501, -180.3501) -> (138.8501, -180.3501)
  line L1721 (138.8501, -180.3501) -> (138.8501, -177.3501)
  line L1722 (138.8501, -177.3501) -> (135.8501, -177.3501)
  line L1723 (135.8501, -177.3501) -> (135.8501, -180.3501)
  line L1724 (135.8501, -180.3501) -> (132.8501, -180.3501)
  line L1725 (132.8501, -180.3501) -> (132.8501, -177.3501)
  line L1726 (132.8501, -177.3501) -> (129.8501, -177.3501)
  line L1727 (129.8501, -177.3501) -> (129.8501, -180.3501)
  line L1728 (129.8501, -180.3501) -> (126.8501, -180.3501)
  line L1729 (126.8501, -180.3501) -> (126.8501, -177.3501)
  line L1730 (126.8501, -177.3501) -> (123.8501, -177.3501)
  line L1731 (123.8501, -177.3501) -> (123.8501, -180.3501)
  line L1732 (123.8501, -180.3501) -> (120.8501, -180.3501)
  line L1733 (120.8501, -180.3501) -> (120.8501, -177.3501)
  line L1734 (120.8501, -177.3501) -> (117.8501, -177.3501)
  line L1735 (117.8501, -177.3501) -> (117.8501, -180.3501)
  line L1736 (117.8501, -180.3501) -> (114.8501, -180.3501)
  line L1737 (114.8501, -180.3501) -> (114.8501, -177.3501)
  line L1738 (114.8501, -177.3501) -> (111.8501, -177.3501)
  line L1739 (111.8501, -177.3501) -> (111.8501, -180.3501)
  line L1740 (111.8501, -180.3501) -> (108.8501, -180.3501)
  line L1741 (108.8501, -180.3501) -> (108.8501, -177.3501)
  line L1742 (108.8501, -177.3501) -> (105.8501, -177.3501)
  line L1743 (105.8501, -177.3501) -> (105.8501, -180.3501)
  line L1744 (105.8501, -180.3501) -> (102.8501, -180.3501)
  line L1745 (102.8501, -180.3501) -> (102.8501, -177.3501)
  line L1746 (102.8501, -177.3501) -> (99.8501, -177.3501)
  line L1747 (99.8501, -177.3501) -> (99.8501, -180.3501)
  line L1748 (99.8501, -180.3501) -> (96.8501, -180.3501)
  line L1749 (96.8501, -180.3501) -> (96.8501, -177.3501)
  line L1750 (96.8501, -177.3501) -> (93.8501, -177.3501)
  line L1751 (93.8501, -177.3501) -> (93.8501, -180.3501)
  line L1752 (93.8501, -180.3501) -> (90.8501, -180.3501)
  line L1753 (90.8501, -180.3501) -> (90.8501, -177.3501)
  line L1754 (90.8501, -177.3501) -> (87.8501, -177.3501)
  line L1755 (87.8501, -177.3501) -> (87.8501, -180.3501)
  line L1756 (87.8501, -180.3501) -> (84.8501, -180.3501)
  line L1757 (84.8501, -180.3501) -> (84.8501, -177.3501)
  line L1758 (84.8501, -177.3501) -> (81.8501, -177.3501)
  line L1759 (81.8501, -177.3501) -> (81.8501, -180.3501)
  line L1760 (81.8501, -180.3501) -> (78.8501, -180.3501)
  line L1761 (78.8501, -180.3501) -> (78.8501, -177.3501)
  line L1762 (78.8501, -177.3501) -> (75.8501, -177.3501)
  line L1763 (75.8501, -177.3501) -> (75.8501, -180.3501)
  line L1764 (75.8501, -180.3501) -> (72.8501, -180.3501)
  line L1765 (72.8501, -180.3501) -> (72.8501, -177.3501)
  line L1766 (72.8501, -177.3501) -> (69.8501, -177.3501)
  line L1767 (69.8501, -177.3501) -> (69.8501, -180.3501)
  line L1768 (69.8501, -180.3501) -> (66.8501, -180.3501)
  line L1769 (66.8501, -180.3501) -> (66.8501, -177.3501)
  line L1770 (66.8501, -177.3501) -> (63.8501, -177.3501)
  line L1771 (63.8501, -177.3501) -> (63.8501, -180.3501)
  line L1772 (63.8501, -180.3501) -> (60.8501, -180.3501)
  line L1773 (60.8501, -180.3501) -> (60.8501, -177.3501)
  line L1774 (60.8501, -177.3501) -> (57.85, -177.3501)
  line L1775 (57.85, -177.3501) -> (57.85, -180.3501)
  line L1776 (57.85, -180.3501) -> (54.85, -180.3501)
  line L1777 (54.85, -180.3501) -> (54.85, -177.3501)
  line L1778 (54.85, -177.3501) -> (51.85, -177.3501)
  line L1779 (51.85, -177.3501) -> (51.85, -180.3501)
  line L1780 (51.85, -180.3501) -> (48.85, -180.3501)
  line L1781 (48.85, -180.3501) -> (48.85, -177.3501)
  line L1782 (48.85, -177.3501) -> (45.85, -177.3501)
  line L1783 (45.85, -177.3501) -> (45.85, -180.3501)
  line L1784 (45.85, -180.3501) -> (42.85, -180.3501)
  line L1785 (42.85, -180.3501) -> (42.85, -177.3501)
  line L1786 (42.85, -177.3501) -> (39.85, -177.3501)
  line L1787 (39.85, -177.3501) -> (39.85, -180.3501)
  line L1788 (39.85, -180.3501) -> (36.85, -180.3501)
  line L1789 (36.85, -180.3501) -> (36.85, -177.3501)
  line L1790 (36.85, -177.3501) -> (33.85, -177.3501)
  line L1791 (33.85, -177.3501) -> (33.85, -180.3501)
  line L1792 (33.85, -180.3501) -> (30.85, -180.3501)
  line L1793 (30.85, -180.3501) -> (30.85, -177.3501)
  line L1794 (30.85, -177.3501) -> (27.85, -177.3501)
  line L1795 (27.85, -177.3501) -> (27.85, -180.3501)
  line L1796 (27.85, -180.3501) -> (24.85, -180.3501)
  line L1797 (24.85, -180.3501) -> (24.85, -177.3501)
  line L1798 (24.85, -177.3501) -> (21.85, -177.3501)
  line L1799 (21.85, -177.3501) -> (21.85, -180.3501)
  line L1800 (21.85, -180.3501) -> (18.85, -180.3501)
  line L1801 (18.85, -180.3501) -> (18.85, -177.3501)
  line L1802 (18.85, -177.3501) -> (15.85, -177.3501)
  line L1803 (15.85, -177.3501) -> (15.85, -180.3501)
  line L1804 (15.85, -180.3501) -> (11.1, -180.3501)
  line L1805 (11.1, -180.3501) -> (11.1, -177.3501)
  line L1806 (11.1, -177.3501) -> (9.35, -177.3501)
  line L1807 (9.35, -177.3501) -> (9.35, -176.6001)
  line L1808 (9.35, -176.6001) -> (6.35, -176.6001)
  line L1809 (6.35, -176.6001) -> (6.35, -172.8501)
  line L1810 (6.35, -172.8501) -> (9.35, -172.8501)
  line L1811 (9.35, -172.8501) -> (9.35, -169.8501)
  line L1812 (9.35, -169.8501) -> (6.35, -169.8501)
  line L1813 (6.35, -169.8501) -> (6.35, -166.8501)
  line L1814 (6.35, -166.8501) -> (9.35, -166.8501)
  line L1815 (9.35, -166.8501) -> (9.35, -163.8501)
  line L1816 (9.35, -163.8501) -> (6.35, -163.8501)
  line L1817 (6.35, -163.8501) -> (6.35, -160.8501)
  line L1818 (6.35, -160.8501) -> (9.35, -160.8501)
  line L1819 (9.35, -160.8501) -> (9.35, -157.8501)
  line L1820 (9.35, -157.8501) -> (6.35, -157.8501)
  line L1821 (6.35, -157.8501) -> (6.35, -154.8501)
  line L1822 (6.35, -154.8501) -> (9.35, -154.8501)
  line L1823 (9.35, -154.8501) -> (9.35, -151.8501)
  line L1824 (9.35, -151.8501) -> (6.35, -151.8501)
  line L1825 (6.35, -151.8501) -> (6.35, -148.8501)
  line L1826 (6.35, -148.8501) -> (9.35, -148.8501)
  line L1827 (9.35, -148.8501) -> (9.35, -145.8501)
  line L1828 (9.35, -145.8501) -> (6.35, -145.8501)
  line L1829 (6.35, -145.8501) -> (6.35, -142.8501)
  line L1830 (6.35, -142.8501) -> (9.35, -142.8501)
  line L1831 (9.35, -142.8501) -> (9.35, -139.8501)
  line L1832 (9.35, -139.8501) -> (6.35, -139.8501)
  line L1833 (6.35, -139.8501) -> (6.35, -136.8501)
  line L1834 (6.35, -136.8501) -> (9.35, -136.8501)
  line L1835 (9.35, -136.8501) -> (9.35, -133.8501)
  line L1836 (9.35, -133.8501) -> (6.35, -133.8501)
  line L1837 (6.35, -133.8501) -> (6.35, -130.8501)
  line L1838 (6.35, -130.8501) -> (9.35, -130.8501)
  line L1839 (9.35, -130.8501) -> (9.35, -127.8501)
  line L1840 (9.35, -127.8501) -> (6.35, -127.8501)
  line L1841 (6.35, -127.8501) -> (6.35, -124.8501)
  line L1842 (6.35, -124.8501) -> (9.35, -124.8501)
  line L1843 (9.35, -124.8501) -> (9.35, -121.8501)
  line L1844 (9.35, -121.8501) -> (6.35, -121.8501)
  line L1845 (6.35, -121.8501) -> (6.35, -118.8501)
  line L1846 (6.35, -118.8501) -> (9.35, -118.8501)
  line L1847 (9.35, -118.8501) -> (9.35, -115.8501)
  line L1848 (9.35, -115.8501) -> (6.35, -115.8501)
  line L1849 (6.35, -115.8501) -> (6.35, -112.8501)
  line L1850 (6.35, -112.8501) -> (9.35, -112.8501)
  line L1851 (9.35, -112.8501) -> (9.35, -109.8501)
  line L1852 (9.35, -109.8501) -> (6.35, -109.8501)
  line L1853 (6.35, -109.8501) -> (6.35, -106.8501)
  line L1854 (6.35, -106.8501) -> (9.35, -106.8501)
  line L1855 (9.35, -106.8501) -> (9.35, -103.8501)
  line L1856 (9.35, -103.8501) -> (6.35, -103.8501)
  line L1857 (6.35, -103.8501) -> (6.35, -100.8501)
  line L1858 (6.35, -100.8501) -> (9.35, -100.8501)
  line L1859 (9.35, -100.8501) -> (9.35, -97.8501)
  line L1860 (9.35, -97.8501) -> (6.35, -97.8501)
  line L1861 (6.35, -97.8501) -> (6.35, -94.8501)
  line L1862 (6.35, -94.8501) -> (9.35, -94.8501)
  line L1863 (9.35, -94.8501) -> (9.35, -91.8501)
  line L1864 (9.35, -91.8501) -> (6.35, -91.8501)
  line L1865 (6.35, -91.8501) -> (6.35, -88.8501)
  line L1866 (6.35, -88.8501) -> (9.35, -88.8501)
  line L1867 (9.35, -88.8501) -> (9.35, -85.8501)
  line L1868 (9.35, -85.8501) -> (6.35, -85.8501)
  line L1869 (6.35, -85.8501) -> (6.35, -82.8501)
  line L1870 (6.35, -82.8501) -> (9.35, -82.8501)
  line L1871 (9.35, -82.8501) -> (9.35, -79.8501)
  line L1872 (9.35, -79.8501) -> (6.35, -79.8501)
  line L1873 (6.35, -79.8501) -> (6.35, -76.8501)
  line L1874 (6.35, -76.8501) -> (9.35, -76.8501)
  line L1875 (9.35, -76.8501) -> (9.35, -73.8501)
  line L1876 (9.35, -73.8501) -> (6.35, -73.8501)
  line L1877 (6.35, -73.8501) -> (6.35, -70.8501)